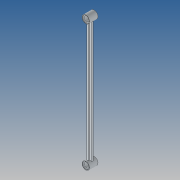
# Autodesk Inventor part: 2739a-Black
Saved by Autodesk Inventor 2022.2 (Build 262287000, 287)
## iProperties
Created: 2014-08-11
Part Number: 2739a-Black
Material: ABS Plastic
Document SubType Name: Modeling
Designer: D. Kohfeld
Mass: 0.550153 g
Surface Area: 10.3816 cm^2
Volume: 0.519012 cm^3
Density: 1.06 g/cm^3
Appearance: LtBluishGray
Description: Link 1 x 6
Author: D. Kohfeld
Autodesk Inventor part; units mm, degrees
ref_plane "YZ Plane" through (0, 0, 0) normal (1, 0, 0) x (0, 1, 0)
ref_plane "XZ Plane" through (0, 0, 0) normal (0, 1, 0) x (-1, 0, 0)
ref_plane "XY Plane" through (0, 0, 0) normal (0, 0, 1) x (1, 0, 0)
sketch "Sketch2" plane through (0, 0, 0) normal (0, 1, 0) x (-1, 0, 0)
  circle A0 centre (0, 0) radius 2.4 construction
  line L0 (-0.8, 2.2627) -> (-0.8, 0.8)
  line L1 (-0.8, 0.8) -> (-2.2627, 0.8)
  line L2 (-2.2627, -0.8) -> (-0.8, -0.8)
  line L3 (-0.8, -0.8) -> (-0.8, -2.2627)
  line L4 (0.8, -2.2627) -> (0.8, -0.8)
  line L5 (0.8, -0.8) -> (2.2627, -0.8)
  line L6 (2.2627, 0.8) -> (0.8, 0.8)
  line L7 (0.8, 0.8) -> (0.8, 2.2627)
  arc A1 (0.8, 2.2627) -> (-0.8, 2.2627) centre (0, 0) ccw
  arc A2 (-2.2627, 0.8) -> (-2.2627, -0.8) centre (0, 0) ccw
  arc A3 (-0.8, -2.2627) -> (0.8, -2.2627) centre (0, 0) ccw
  arc A4 (2.2627, -0.8) -> (2.2627, 0.8) centre (0, 0) ccw
  dimension "d1" = 4.8
  dimension "d0" = 1.6
  constraints: 16 end point, 8 point on circle, 7 equal length, 4 centre point, 4 perpendicular, 3 parallel, 1 coincident, 1 vertical, 14 other
  measures "d0" distance between parallel lines of L7 L0
extrude "Extrusion1" add sketch "Sketch2" along normal mid plane 120
sketch "Sketch3" plane through (0, 0, 0) normal (0, 0, 1) x (1, 0, 0)
  line L0 (0.8, 60) -> (-0.8, 60) projected
  line L1 (-0.8, -60) -> (0.8, -60) projected
  circle A0 centre (0, 60) radius 3.6
  circle A1 centre (0, 60) radius 2.4
  circle A2 centre (0, -60) radius 3.6
  circle A3 centre (0, -60) radius 2.4
  point P0 (0, 0)
  dimension "d4" = 7.2
  dimension "d5" = 4.8
  constraints: 4 centre point, 2 coincident, 2 equal radius, 2 midpoint
  measures "d4" diameter of A0
  measures "d5" diameter of A1
extrude "Extrusion2" add sketch "Sketch3" along normal mid plane 8 contours A0 | A1 | A2 | A3
sketch "Sketch4" plane through (0, 60, -4) normal (0, 0, -1) x (-1, 0, 0)
  circle A0 centre (0, 0) radius 3.6 projected
  circle A1 centre (0, 0) radius 2.4
  circle A2 centre (0, -120) radius 3.6 projected
  circle A3 centre (0, -120) radius 2.4
  point P0 (0, -3.6)
  point P1 (0, -60)
  dimension "d10" = 4.8
  constraints: 2 centre point, 2 coincident, 1 equal radius, 1 vertical alignment
  measures "d10" diameter of A1
extrude "Extrusion4" cut sketch "Sketch4" against normal through all contours A1 | A3
sketch "Skizze6" plane through (0, 60, -4) normal (0, 0, -1) x (-1, 0, 0)
  circle A0 centre (0, 0) radius 2.4 projected
  circle A1 centre (0, 0) radius 3.6 projected
  circle A2 centre (0, 0) radius 3.2
  point P0 (0, -60)
  dimension "d26" = 6.4
  constraints: 1 centre point, 1 coincident
  measures "d26" diameter of A2
extrude "Extrusion5" cut sketch "Skizze6" against normal blind 0.8 contours A2
pattern_circular "Circular Pattern1" count 2 over 360 about axis through (0, 0, 0) along (0, -1, 0) of "Extrusion5"
pattern_linear "Rectangular Pattern1" count 2 spacing 120 along (0, -1, 0) of "Circular Pattern1", "Extrusion5"
equation "\"d1\" = kd"
equation "\"d0\" = axlet"
equation "\"d2\" = 15 * lu"
equation "\"d4\" = tlad"
equation "\"d5\" = tpd"
equation "\"d6\" = lu"
equation "\"d10\" = tpd"
equation "\"d11\" = tsl"
equation "\"d26\" = tsd"
equation "\"d27\" = tsl"
equation "\"d25\" = 15 * lu"
equation "\"kd\" = 4.8"
equation "\"axlet\" = 1.6"
equation "\"lu\" = 8"
equation "\"tlad\" = 7.2"
equation "\"tpd\" = 4.8"
equation "\"tsl\" = 0.8"
equation "\"tsd\" = 6.4"
body "Solid1"
